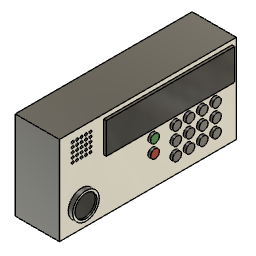
ece1895_bopit_exterior (Autodesk Fusion 360 design; units mm, degrees)
Autodesk Fusion 360 part; units mm, degrees
sketch "Sketch1" plane through (0, 0, 0) normal (1, 0, 0) x (0, 1, 0)
  line L0 (0, 0) -> (200, 0)
  line L1 (200, 0) -> (200, 100)
  line L2 (200, 100) -> (0, 100)
  line L3 (0, 100) -> (0, 0)
  constraint horizontal L0
  constraint vertical L1
  constraint horizontal L2
  constraint vertical L3
  constraint coincident L0.start L3.end
extrude "Extrude1" add sketch "Sketch1" along normal blind 50
sketch "Sketch2" plane through (50, 0, 0) normal (1, 0, 0) x (0, 1, 0)
  line L0 (0, 100) -> (0, 0)
  line L1 (0, 0) -> (200, 0)
  line L2 (200, 0) -> (200, 100)
  line L3 (200, 100) -> (0, 100)
shell "Shell1" thickness 5 removed faces 1 at (0, 66.6667, 66.6667)
sketch "Sketch3" plane through (50, 0, 0) normal (1, 0, 0) x (0, 1, 0)
  circle A0 centre (175, 50) radius 5
  line L0 (50, 60) -> (50, 95)
  line L1 (200, 0) -> (200, 100)
  circle A1 centre (130, 20) radius 5
  circle A2 centre (175, 20) radius 5
  circle A3 centre (25, 25) radius 15
  line L2 (195, 95) -> (195, 60)
  circle A4 centre (145, 20) radius 5
  circle A5 centre (145, 35) radius 5
  circle A6 centre (160, 50) radius 5
  circle A7 centre (105, 35) radius 5
  line L3 (0, 0) -> (200, 0)
  circle A8 centre (130, 50) radius 5
  line L4 (200, 100) -> (0, 100)
  line L5 (195, 60) -> (50, 60)
  circle A9 centre (160, 20) radius 5
  circle A10 centre (130, 35) radius 5
  circle A11 centre (105, 50) radius 5
  circle A12 centre (160, 35) radius 5
  circle A13 centre (175, 35) radius 5
  circle A14 centre (145, 50) radius 5
  line L6 (50, 95) -> (195, 95)
  line L7 (0, 100) -> (0, 0)
  circle A15 centre (25, 25) radius 12.5
  point P0 (30, 85)
  point P1 (30, 70)
  point P2 (30, 90)
  point P3 (15, 85)
  point P4 (25, 90)
  point P5 (30, 75)
  point P6 (15, 70)
  point P7 (35, 85)
  point P8 (20, 85)
  point P9 (20, 80)
  point P10 (15, 80)
  point P11 (35, 80)
  point P12 (25, 85)
  point P13 (15, 75)
  point P14 (20, 75)
  point P15 (35, 90)
  point P16 (20, 90)
  point P17 (25, 75)
  point P18 (35, 75)
  point P19 (30, 80)
  point P20 (15, 90)
  point P21 (25, 80)
  point P22 (25, 70)
  point P23 (20, 70)
  point P24 (35, 70)
  dimension "d8" = 10
  dimension "d9" = 10
  dimension "d10" = 10
  dimension "d11" = 30
  dimension "d21" = 25
  constraint horizontal L3
  constraint vertical L1
  constraint horizontal L4
  constraint vertical L7
  constraint coincident L3.start L7.end
  constraint horizontal L6
  constraint vertical L2
  constraint horizontal L5
  constraint vertical L0
  constraint concentric A3 A15
  measures "d8" diameter of A6
  measures "d9" diameter of A14
  measures "d10" diameter of A8
  measures "d11" diameter of A3
  measures "d21" diameter of A15
hole "Hole1" at (50, 35, 90) at (50, 30, 90) at (50, 25, 90) at (50, 20, 90) at (50, 15, 90) at (50, 15, 85) at (50, 15, 80) at (50, 15, 75) at (50, 15, 70) at (50, 20, 70) at (50, 20, 75) at (50, 20, 80) at (50, 25, 85) at (50, 20, 85) at (50, 25, 80) at (50, 25, 75) at (50, 25, 70) at (50, 30, 70) at (50, 30, 75) at (50, 30, 80) at (50, 30, 85) at (50, 35, 85) at (50, 35, 80) at (50, 35, 75) at (50, 35, 70) direction (-1, 0, 0) diameter 3 depth 5 tip angle 180
extrude "Extrude2" add sketch "Sketch3" along normal blind 3 contours L0 L2 L5 L6
extrude "Extrude3" add sketch "Sketch3" along normal blind 3 contours A11
extrude "Extrude4" add sketch "Sketch3" along normal blind 3 contours A0 | A1 | A2 | A4 | A5 | A6 | A7 | A8 | A9 | A10 | A12 | A13 | A14
extrude "Extrude5" add sketch "Sketch3" along normal blind 5 contours A3
extrude "Extrude6" add sketch "Sketch3" along normal blind 3 contours A15
